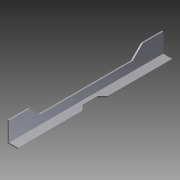
# Autodesk Inventor part: 8 ball  frame bottom L
Saved by Autodesk Inventor 2012 (Build 160160000, 160)
## iProperties
Created: 2013-10-18
Part Number: 8 ball  frame bottom L
Material: Default
Document SubType Name: Modeling
Designer: Bryce
Density: 1 g/cm^3
Author: Bryce
Autodesk Inventor part; units mm, degrees
ref_plane "YZ Plane" through (0, 0, 0) normal (1, 0, 0) x (0, 1, 0)
ref_plane "XZ Plane" through (0, 0, 0) normal (0, 1, 0) x (-1, 0, 0)
ref_plane "XY Plane" through (0, 0, 0) normal (0, 0, 1) x (1, 0, 0)
sketch "Sketch1" plane through (0, 0, 0) normal (0, 0, 1) x (1, 0, 0)
  line L0 (0, 0) -> (25.3902, 0)
  line L1 (25.3902, 0) -> (25.3902, 3.175)
  line L2 (3.175, 50.8) -> (0, 50.8)
  line L3 (0, 50.8) -> (0, 0)
  line L4 (3.175, 50.8) -> (3.175, 3.175)
  line L5 (3.175, 3.175) -> (25.3902, 3.175)
  dimension "d0" = 50.8
  dimension "d1" = 25.3902
  dimension "d2" = 3.175
  dimension "d3" = 3.175
  constraints: 12 end point, 2 parallel, 1 horizontal, 1 perpendicular
  measures "d0" distance of L2.end L0.start
  measures "d1" distance of L0.start L0.end
  measures "d2" distance between parallel lines of L0 L5
  measures "d3" distance between parallel lines of L3 L4
extrude "Extrusion1" add sketch "Sketch1" along normal blind 381
sketch "Sketch2" plane through (0, 0, 0) normal (0, -1, 0) x (1, 0, 0)
  line L0 (0, 0) -> (25.3902, 0) projected
  line L1 (25.3902, 0) -> (25.3902, 381) projected
  line L2 (25.3902, 158.75) -> (12.6902, 171.45)
  line L3 (12.6902, 171.45) -> (12.6902, 209.55)
  line L4 (12.6902, 209.55) -> (25.3902, 222.25)
  dimension "d6" = 12.7
  dimension "d7" = 45
  dimension "d8" = 45
  dimension "d9" = 38.1
  dimension "d10" = 171.45
  constraints: 6 end point, 2 point on line, 1 parallel
  measures "d6" distance between parallel lines of L1 L3
  measures "d7" angle of L4 L3
  measures "d8" angle of L2 L3
  measures "d9" distance of L2.end L3.end
  measures "d10" distance from line of L0 L2.end
extrude "Extrusion2" cut sketch "Sketch2" against normal through all
sketch "Sketch3" plane through (0, 0, 0) normal (-1, 0, 0) x (0, 0, 1)
  line L0 (381, 0) -> (381, 50.8) projected
  line L1 (0, 50.8) -> (381, 50.8) projected
  line L2 (0, 50.8) -> (0, 0) projected
  line L3 (0, 0) -> (381, 0) projected
  line L4 (50.8, 50.8) -> (76.2, 25.4)
  line L5 (76.2, 25.4) -> (304.8, 25.4)
  line L6 (304.8, 25.4) -> (330.2, 50.8)
  dimension "d13" = 25.4
  dimension "d14" = 45
  dimension "d15" = 45
  dimension "d16" = 50.8
  dimension "d17" = 50.8
  constraints: 6 end point, 2 point on line, 1 parallel
  measures "d13" distance between parallel lines of L1 L5
  measures "d14" angle of L5 L4
  measures "d15" angle of L5 L6
  measures "d16" distance from line of L0 L6.end
  measures "d17" distance from line of L4.start L2
extrude "Extrusion3" cut sketch "Sketch3" against normal through all contours L6 L5 L4 L1
equation "\"d2\" = d3"
equation "\"d7\" = d8"
equation "\"d15\" = d14"
equation "\"d17\" = d16"
body "Solid1"
